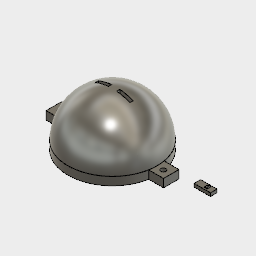
btmbtm - Copy (Autodesk Fusion 360 design; units mm, degrees)
Autodesk Fusion 360 part; units mm, degrees
sketch "Sketch1" plane through (0, 0, 0) normal (0, 1, 0) x (1, 0, 0)
  circle A0 centre (0, 0) radius 25
  circle A1 centre (0, 0) radius 27
  circle A2 centre (0, 0) radius 26
  line L0 (-26.5898, 4.6885) -> (-35.5898, 4.6885)
  line L1 (-26.5898, -4.6885) -> (-35.5898, -4.6885)
  line L2 (-35.5898, 4.6885) -> (-35.5898, -4.6885)
  line L3 (0, 0) -> (26.3565, 0) construction
  line L4 (26.5898, 4.6885) -> (35.5898, 4.6885)
  line L5 (26.5898, -4.6885) -> (35.5898, -4.6885)
  line L6 (35.5898, -4.6885) -> (35.5898, 4.6885)
  line L7 (35.5898, 4.6885) -> (35.5898, -0.3115)
  line L8 (35.5898, -0.3115) -> (31.0898, -0.3115)
  line L9 (-35.5898, 4.6885) -> (-35.5898, -0.3115)
  line L10 (-35.5898, -0.3115) -> (-31.0898, -0.3115)
  circle A3 centre (-31.0898, -0.3115) radius 1.5
  circle A4 centre (31.0898, -0.3115) radius 1.5
extrude "Extrude7" add sketch "Sketch1" along normal blind 5 contours A1 L4 L5 L6 L7 makes body 1
extrude "Extrude10" cut sketch "Sketch1" along normal blind 95 contours A1 L0 L1 L2 L9 bodies 1
extrude "Extrude11" add sketch "Sketch1" along normal blind 5 contours A1 L0 L1 L2 L9 bodies 1 makes body 2
extrude "Extrude12" add sketch "Sketch1" along normal blind 5 contours A1 | A2 bodies 1 2
sketch "Sketch3" plane through (0, 0, 0) normal (1, 0, 0) x (0, 0, -1)
form "Form1" [no effect]
sphere "SpherePrimitive2" add diameter 54 placed x (1, 0, 0) y (0, 0, -1) z (0, 1, 0) at (-0.5647, 0, 72.4609) separate body makes body 3
sketch "Sketch5" plane through (0, 0, 0) normal (1, 0, 0) x (0, 0, -1)
  line L0 (-4.6885, 0) -> (-27, 0)
  line L1 (0, 0) -> (-152.1039, 0)
split_face "SplitFace1" 1 faces at (25.0333, 6.3823, 66.7157) by curves path "Sketch5" along L1 on bodies 3
split_face "SplitFace2" 2 faces at (25.0333, 6.3823, 66.7157) (25.0333, -6.3823, 66.7157) by plane through (0, 0, 0) normal (0, 1, 0) on bodies 3
move_body "Align1" bodies 3 to x (0, 0, 1) y (0, 1, 0) z (-1, 0, 0) at (72.4609, 0, 0.5647)
move_face "MoveFace7" to x (1, 0, 0) y (0, 1, 0) z (0, 0, 1) at (0, 5, 0) 1 faces at (5.7452, 6.3823, 25.598) on bodies 3
move_face "OffsetFaces1" offset -25 1 faces at (-19.8737, 1.4758, 17.9337) on bodies 3
delete_face "DeleteFace1" 1 faces at (1.9723, 4.7389, 0.2049) on bodies 3
sketch "Sketch6" plane through (0, 5, 0) normal (0, -1, 0) x (1, 0, 0)
  circle A0 centre (0, 0) radius 27
  line L0 (0, 0) -> (10.5, 0)
  line L1 (10.5, 0) -> (10.5, -2)
  line L2 (10.5, -2) -> (-10.5, -2)
  line L3 (-10.5, -2) -> (-10.5, 0)
  line L4 (-10.5, 0) -> (0, 0)
  line L5 (-10.5, 0) -> (-2.5, 0)
  line L6 (-2.5, 0) -> (-2.5, -2)
  line L7 (10.5, 0) -> (2.5, 0)
  line L8 (2.5, 0) -> (2.5, -2)
  dimension "d47" = 10.5
  dimension "d48" = 2
  dimension "d49" = 21
  dimension "d50" = 2
  dimension "d51" = 8
  dimension "d52" = 2
  dimension "d53" = 8
  measures "d47" distance of A0.centre L0.end
  measures "d48" distance of L0.end L1.end
  measures "d49" distance of L1.end L2.end
  measures "d50" distance of L2.end L3.end
  measures "d51" distance of L3.end L5.end
  measures "d52" distance of L5.end L6.end
  measures "d53" distance of L0.end L7.end
extrude "Extrude13" cut sketch "Sketch6" against normal blind 30 contours L0 L1 L2 L7 L8 | L2 L3 L4 L5 L6 bodies 3
sketch "Sketch7" plane through (0, 5, 0) normal (0, -1, 0) x (1, 0, 0)
  line L0 (-10.5, -2) -> (-10.5, 0)
  line L1 (-10.5, 0) -> (-2.5, 0)
  line L2 (-2.5, 0) -> (-2.5, -2)
  line L3 (-2.5, -2) -> (-10.5, -2)
  line L4 (2.5, -2) -> (2.5, 0)
  line L5 (2.5, 0) -> (10.5, 0)
  line L6 (10.5, 0) -> (10.5, -2)
  line L7 (10.5, -2) -> (2.5, -2)
  circle A0 centre (0, 0) radius 27
  line L8 (-2.5, 0) -> (2.5, 0)
  line L9 (-2.5, -2) -> (2.5, -2)
extrude "Extrude14" cut sketch "Sketch7" against normal blind 22 contours L2 L4 L8 L9 bodies 3
sketch "Sketch8" plane through (0, 5, 0) normal (0, -1, 0) x (1, 0, 0)
  circle A0 centre (0, 0) radius 27
  line L0 (10.5, -2) -> (-10.5, -2)
  line L1 (-10.5, -2) -> (-10.5, 0)
  line L2 (-10.5, 0) -> (10.5, 0)
  line L3 (10.5, 0) -> (10.5, -2)
  line L4 (10.5, 0) -> (3.5, 0)
  line L5 (-10.5, 0) -> (-3.5, 0)
  line L6 (-3.5, 0) -> (-3.5, 6)
  line L7 (3.5, 0) -> (3.5, 6)
  line L8 (3.5, 6) -> (-3.5, 6)
  dimension "d62" = 7
  dimension "d63" = 7
  dimension "d64" = 6
  dimension "d65" = 6
  measures "d62" distance of L2.end L4.end
  measures "d63" distance of L1.end L5.end
  measures "d64" distance of L5.end L6.end
  measures "d65" distance of L4.end L7.end
extrude "Extrude15" cut sketch "Sketch8" against normal blind 15 contours L2 L6 L7 L8 bodies 3
sketch "Sketch9" plane through (0, 5, 0) normal (0, -1, 0) x (1, 0, 0)
  line L0 (-3.5, 0) -> (-3.5, 6)
  line L1 (-3.5, 6) -> (3.5, 6)
  line L2 (3.5, 6) -> (3.5, 0)
  line L3 (3.5, 0) -> (10.5, 0)
  line L4 (10.5, 0) -> (10.5, -2)
  line L5 (10.5, -2) -> (-10.5, -2)
  line L6 (-10.5, -2) -> (-10.5, 0)
  line L7 (-10.5, 0) -> (-3.5, 0)
  circle A0 centre (0, 0) radius 27
  line L8 (-10.5, -2) -> (-3.5, -2)
  line L9 (10.5, -2) -> (3.5, -2)
  line L10 (3.5, -2) -> (3.5, -3)
  line L11 (-3.5, -2) -> (-3.5, -3)
  line L12 (-3.5, -3) -> (3.5, -3)
  dimension "d68" = 7
  dimension "d69" = 7
  dimension "d70" = 1
  dimension "d71" = 1
  measures "d68" distance of L5.end L8.end
  measures "d69" distance of L4.end L9.end
  measures "d70" distance of L9.end L10.end
  measures "d71" distance of L8.end L11.end
extrude "Extrude16" cut sketch "Sketch9" against normal blind 15 contours L5 L10 L11 L12 bodies 3
sketch "Sketch10" plane through (0, 0, 6) normal (0, 0, -1) x (-1, 0, 0)
  line L0 (-3.5, 5) -> (3.5, 5)
  line L1 (3.5, 5) -> (3.5, 20)
  line L2 (3.5, 20) -> (-3.5, 20)
  line L3 (-3.5, 20) -> (-3.5, 5)
  line L4 (3.5, 5, 9) -> (1.5, 5, 9)
  line L5 (-3.5, 5, 9) -> (-1.5, 5, 9)
  line L6 (10.5, 5, 8) -> (7.5, 5, 8)
  line L7 (7.5, 5, 8) -> (7.5, 8, 8)
  line L8 (7.5, 8, 8) -> (9.5, 8, 8)
  line L9 (9.5, 8, 8) -> (9.5, 10, 8)
  line L10 (9.5, 10, 8) -> (7.5, 10, 8)
  line L11 (7.5, 10, 8) -> (7.5, 8, 8)
  point P0 (3.5, 5)
  point P1 (-3.5, 5)
  point P2 (10.5, 5)
  dimension "d74" = 2
  dimension "d75" = 2
  dimension "d76" = 3
  dimension "d79" = 3
  dimension "d80" = 2
  dimension "d81" = 2
  dimension "d82" = 2
extrude "Extrude17" cut sketch "Sketch10" along normal blind 2 contours L8 L9 L10 L11 in plane through (0, 0, -2) normal (0, 0, -1) bodies 3
sketch "Sketch11" plane through (-9.5, 0, 0) normal (1, 0, 0) x (0, 0, -1)
  line L0 (2, 10) -> (2, 8)
  line L1 (2, 8) -> (4, 8)
  line L2 (4, 8) -> (4, 10)
  line L3 (4, 10) -> (2, 10)
  line L4 (2, 5, -1) -> (2, 29.7942, -1)
  line L5 (2, 8, 0) -> (2, 8, -1)
  line L6 (0.8014, -0.3321) -> (0.6162, -0.3321)
  line L7 (0.6162, -0.3321) -> (1.1867, -0.3321)
  line L8 (2, 5, 20) -> (2, 5, 19)
  line L9 (1.1072, -0.4689) -> (1.2319, -0.4689)
  line L10 (2, 5, 19) -> (2, 8, 19)
  line L11 (2, 8, 19) -> (2, 8, 17)
  line L12 (2, 8, 19) -> (2, 10, 19)
  line L13 (2, 10, 19) -> (2, 10, 17)
  line L14 (2, 10, 17) -> (2, 8, 17)
  point P0 (2, 5)
  dimension "d87" = 2
  dimension "d88" = 2
  dimension "d89" = 2
  measures "d87" distance of L0.end L1.start
  measures "d88" distance of L0.end L0.start
  measures "d89" distance of L0.start L3.end
extrude "Extrude18" cut sketch "Sketch11" along normal blind 2 contours L11 L12 L13 L14 in plane through (-9.5, 0, -2) normal (0, 0, -1) bodies 3
sketch "Sketch12" plane through (0, 0, 0) normal (0, 1, 0) x (1, 0, 0)
  line L0 (44.3552, 8.9685) -> (54.3552, 8.9685)
  line L1 (54.3552, 8.9685) -> (54.3552, 4.9685)
  line L2 (54.3552, 4.9685) -> (44.3552, 4.9685)
  line L3 (44.3552, 4.9685) -> (44.3552, 8.9685)
  dimension "d92" = 10
  dimension "d93" = 4
  measures "d92" distance of L0.start L0.end
  measures "d93" distance of L0.start L2.end
extrude "Extrude19" add sketch "Sketch12" along normal blind 2 separate body makes body 4
sketch "Sketch13" plane through (0, 2, 0) normal (0, 1, 0) x (-1, 0, 0)
  line L0 (-44.3552, -4.9685) -> (-54.3552, -4.9685)
  line L1 (-54.3552, -4.9685) -> (-54.3552, -8.9685)
  line L2 (-54.3552, -8.9685) -> (-44.3552, -8.9685)
  line L3 (-44.3552, -8.9685) -> (-44.3552, -4.9685)
  line L4 (-54.3552, -8.9685) -> (-51.3552, -8.9685)
  line L5 (-54.3552, -4.9685) -> (-51.3552, -4.9685)
  line L6 (-51.3552, -4.9685) -> (-51.3552, -5.9685)
  line L7 (-51.3552, -8.9685) -> (-51.3552, -7.9685)
  line L8 (-51.3552, -7.9685) -> (-49.3552, -7.9685)
  line L9 (-51.3552, -5.9685) -> (-49.3552, -5.9685)
  line L10 (-49.3552, -7.9685) -> (-49.3552, -5.9685)
  line L11 (-51.3552, -7.9685) -> (-51.3552, -5.9685)
  dimension "d97" = 3
  dimension "d100" = 2
  dimension "d101" = 2
  dimension "d102" = 2
  measures "d97" distance of L0.end L5.end
  measures "d100" distance of L7.end L8.end
  measures "d101" distance of L6.end L9.end
  measures "d102" distance of L8.end L9.end
extrude "Extrude20" add sketch "Sketch13" along normal blind 1 contours L8 L9 L10 L11 bodies 4
sketch "Sketch14" plane through (0, 0, -5.9685) normal (0, 0, 1) x (1, 0, 0)
  line L0 (49.3552, 2) -> (51.3552, 2)
  line L1 (51.3552, 2) -> (51.3552, 3)
  line L2 (51.3552, 3) -> (49.3552, 3)
  line L3 (49.3552, 3) -> (49.3552, 2)
  line L4 (51.3552, 3) -> (49.3552, 2)
extrude "Extrude21" cut sketch "Sketch14" against normal blind 2 contours L2 L3 L4 bodies 4
copy_body "CopyPasteBodies1" bodies 4 makes body 5
copy_body "CopyPasteBodies2" bodies 4 makes body 6
